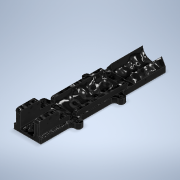
# Autodesk Inventor part: kicker_plate_modified
Saved by Autodesk Inventor 2020 (Build 240168000, 168)
## iProperties
Created: 2019-08-27
Part Number: kicker_plate_modified
Material: PET Plastic
Document SubType Name: Modeling
Designer: felip
Density: 1.541 g/cm^3
Appearance: Black
Author: felip
Autodesk Inventor part; units mm, degrees
ref_plane "YZ Plane" through (0, 0, 0) normal (1, 0, 0) x (0, 1, 0)
ref_plane "XZ Plane" through (0, 0, 0) normal (0, 1, 0) x (-1, 0, 0)
ref_plane "XY Plane" through (0, 0, 0) normal (0, 0, 1) x (1, 0, 0)
sketch "Sketch1" plane through (0, 0, 0) normal (0, 1, 0) x (-1, 0, 0)
  line L0 (0, 0) -> (29, 0)
  line L1 (29, 0) -> (29, -100)
  line L2 (29, -100) -> (0, -100)
  line L3 (0, -100) -> (0, 0)
  dimension "d0" = 29
  dimension "d1" = 100
  constraints: 8 end point, 2 parallel, 1 horizontal, 1 perpendicular
  measures "d0" distance of L1.end L2.end
  measures "d1" distance of L0.end L1.end
extrude "Extrusion1" add sketch "Sketch1" along normal blind 6
ref_plane "Work Plane1" through (-29, 0, -7) normal (0, 0, 1) x (1, 0, 0)
sketch "Sketch2" plane through (-29, 0, -7) normal (0, 0, 1) x (1, 0, 0)
  line L0 (0, 0) -> (29, 0) projected
  line L1 (29, 0) -> (29, 6) projected
  line L2 (0, 6) -> (29, 6) projected
  line L3 (0, 0) -> (0, 6) projected
  line L4 (29, 0) -> (0, 0) construction
  line L5 (14.5, 0) -> (14.5, 12.5) construction
  circle A0 centre (14.5, 12.5) radius 10.75
  point P0 (23.0623, 6)
  point P1 (5.9377, 6)
  dimension "d5" = 12.5
  dimension "d6" = 21.5
  constraints: 2 end point, 1 centre point, 1 coincident, 1 midpoint, 1 vertical
  measures "d5" distance of L5.start L5.end
  measures "d6" diameter of A0
extrude "Extrusion2" cut sketch "Sketch2" against normal blind 51.8 contours A0 L2 | L2 A0
sketch "Sketch9" plane through (0, 6, 0) normal (0, 1, 0) x (1, 0, 0)
  line L0 (-5.9377, 58.8) -> (-5.9377, 7) projected
  line L1 (-5.9377, 7) -> (-23.0623, 7) projected
  line L2 (-23.0623, 7) -> (-23.0623, 58.8) projected
  line L3 (-23.0623, 58.8) -> (-5.9377, 58.8) projected
  line L4 (-29, 100) -> (-29, 0) projected
  line L5 (-29, 0) -> (0, 0) projected
  line L6 (0, 0) -> (0, 100) projected
  line L7 (0, 100) -> (-29, 100) projected
  line L8 (-29, 100) -> (-29, 0) projected
  line L9 (0, 0) -> (0, 100) projected
  line L10 (-29, 100) -> (0, 100)
  line L11 (0, 100) -> (0, 66)
  line L12 (0, 66) -> (-29, 66)
  line L13 (-29, 66) -> (-29, 100)
  dimension "d60" = 34
  constraints: 8 end point, 2 parallel, 1 horizontal, 1 perpendicular, 1 point on line
  measures "d60" distance between parallel lines of L7 L12
extrude "Extrusion7" add sketch "Sketch9" along normal blind 6.75 contours L7 L6 L12 L4
sketch "Sketch3" plane through (0, 0, -100) normal (0, 0, -1) x (-1, 0, 0)
  line L0 (0, 0) -> (29, 0) projected
  line L1 (29, 0) -> (29, 12.75) projected
  line L2 (0, 0) -> (0, 12.75) projected
  line L3 (0, 0) -> (29, 0) construction
  line L4 (14.5, 0) -> (14.5, 12.5) construction
  circle A0 centre (14.5, 12.5) radius 10
  line L5 (0, 12.75) -> (29, 12.75) projected
  dimension "d9" = 12.5
  dimension "d10" = 20
  constraints: 2 end point, 1 centre point, 1 coincident, 1 midpoint, 1 vertical
  measures "d9" distance of L4.start L4.end
  measures "d10" diameter of A0
extrude "Extrusion3" cut sketch "Sketch3" against normal blind 34 contours L5 A0 | A0 L5
sketch "Sketch4" plane through (0, 0, 0) normal (0, -1, 0) x (1, 0, 0)
  line L0 (0, -100) -> (-29, -100) projected
  line L1 (0, 0) -> (0, -100) projected
  line L2 (-29, 0) -> (0, 0) projected
  line L3 (-29, -100) -> (-29, 0) projected
  point P0 (-24, -3)
  point P1 (-5, -3)
  point P2 (-24, -63)
  point P3 (-5, -63)
  dimension "d13" = 3
  dimension "d14" = 5
  dimension "d15" = 3
  dimension "d16" = 5
  dimension "d24" = 5
  dimension "d25" = 63
  dimension "d26" = 5
  dimension "d27" = 63
  measures "d13" distance from line of L2 point (-24, -3)
  measures "d14" distance from line of L3 point (-24, -3)
  measures "d15" distance from line of L2 point (-5, -3)
  measures "d16" distance from line of L1 point (-5, -3)
  measures "d24" distance from line of L3 point (-24, -63)
  measures "d25" distance from line of L2 point (-24, -63)
  measures "d26" distance from line of L1 point (-5, -63)
  measures "d27" distance from line of point (-5, -63) L2
hole "Hole1" at (-24, 0, -3) at (-5, 0, -3) at (-24, 0, -63) at (-5, 0, -63) direction (0, 1, 0) diameter 3.1 depth 6 counterbore diameter 5.5 counterbore depth 2
move faces "Move1" translate (0, 0, 31) faces at (-19.3333, 2, 0)
sketch "Sketch5" plane through (0, 6, 0) normal (0, 1, 0) x (1, 0, 0)
  circle A0 centre (-24, 63) radius 1.55 projected
  circle A1 centre (-24, 3) radius 1.55 projected
  circle A2 centre (-5, 3) radius 1.55 projected
  circle A3 centre (-5, 63) radius 1.55 projected
  line L0 (-6.9007, 66) -> (-22.0993, 66) projected
  line L1 (-29, 66) -> (-29, -31) projected
  line L2 (-29, -31) -> (0, -31) projected
  line L3 (0, -31) -> (0, 66) projected
  line L4 (-5.9377, 58.8) -> (-5.9377, 7) projected
  line L5 (-5.9377, 7) -> (-23.0623, 7) projected
  line L6 (-23.0623, 7) -> (-23.0623, 58.8) projected
  line L7 (-23.0623, 58.8) -> (-5.9377, 58.8) projected
  line L8 (-29, -31) -> (0, -31) projected
  line L9 (-9.25, -31) -> (-19.75, -31)
  line L10 (-19.75, -31) -> (-19.75, 0)
  line L11 (-19.75, 0) -> (-9.25, 0)
  line L12 (-9.25, 0) -> (-9.25, -31)
  line L13 (0, 66) -> (-6.9007, 66) projected
  line L14 (-22.0993, 66) -> (-29, 66) projected
  point P0 (0, 0)
  point P1 (-14.5, -31)
  point P2 (-9.25, -31)
  dimension "d31" = 10.5
  dimension "d32" = 31
  constraints: 8 end point, 2 midpoint, 2 parallel, 1 horizontal, 1 perpendicular, 1 point on line
  measures "d31" distance of L10.end L11.end
  measures "d32" distance of L9.end L10.end
extrude "Extrusion4" cut sketch "Sketch5" against normal blind 2.95 contours L2 L10 L11 L12
sketch "Sketch6" plane through (0, 6, 0) normal (0, 1, 0) x (1, 0, 0)
  line L0 (-5.9377, 58.8) -> (-5.9377, 7) projected
  line L1 (-5.9377, 7) -> (-23.0623, 7) projected
  line L2 (-23.0623, 7) -> (-23.0623, 58.8) projected
  line L3 (-23.0623, 58.8) -> (-5.9377, 58.8) projected
  line L4 (-19.75, -31) -> (-19.75, 0) projected
  line L5 (-19.75, 0) -> (-9.25, 0) projected
  line L6 (-9.25, 0) -> (-9.25, -31) projected
  line L7 (-9.25, -31) -> (0, -31) projected
  line L8 (0, -31) -> (0, 66) projected
  line L9 (-6.9007, 66) -> (-22.0993, 66) projected
  line L10 (-29, 66) -> (-29, -31) projected
  line L11 (-29, -31) -> (-19.75, -31) projected
  circle A0 centre (-5, 63) radius 1.55 projected
  circle A1 centre (-5, 3) radius 1.55 projected
  circle A2 centre (-24, 3) radius 1.55 projected
  circle A3 centre (-24, 63) radius 1.55 projected
  line L12 (-9.25, -31) -> (0, -31) projected
  line L13 (-2.125, -31) -> (-7.125, -31)
  line L14 (-7.125, -31) -> (-7.125, -11)
  line L15 (-7.125, -11) -> (-2.125, -11)
  line L16 (-2.125, -11) -> (-2.125, -31)
  line L17 (-21.875, -31) -> (-26.875, -31)
  line L18 (-26.875, -31) -> (-26.875, -11)
  line L19 (-26.875, -11) -> (-21.875, -11)
  line L20 (-21.875, -11) -> (-21.875, -31)
  line L21 (0, 66) -> (-6.9007, 66) projected
  line L22 (-22.0993, 66) -> (-29, 66) projected
  line L23 (-19.75, -31) -> (-19.75, 0) projected
  line L24 (-21.875, 0) -> (-19.75, 0)
  line L25 (-19.75, 0) -> (-19.75, -31)
  line L26 (-19.75, -31) -> (-21.875, -31)
  line L27 (-21.875, -31) -> (-21.875, 0)
  line L28 (-9.25, 0) -> (-9.25, -31) projected
  line L29 (-7.125, 0) -> (-9.25, 0)
  line L30 (-9.25, 0) -> (-9.25, -31)
  line L31 (-9.25, -31) -> (-7.125, -31)
  line L32 (-7.125, -31) -> (-7.125, 0)
  point P0 (0, 0)
  point P1 (-4.625, -31)
  point P2 (-24.375, -31)
  point P3 (-26.875, -31)
  point P4 (-2.125, -31)
  dimension "d35" = 5
  dimension "d36" = 20
  dimension "d37" = 5
  dimension "d38" = 20
  constraints: 32 end point, 8 parallel, 4 horizontal, 4 midpoint, 4 perpendicular, 3 point on line
  measures "d35" distance of L14.end L15.end
  measures "d36" distance of L13.end L14.end
  measures "d37" distance of L18.end L19.end
  measures "d38" distance of L17.end L18.end
extrude "Extrusion5" add sketch "Sketch6" along normal blind 14 contours L11 L18 L19 L20 | L14 L15 L16 L7
sketch "Sketch7" plane through (0, 0, 0) normal (0, -1, 0) x (1, 0, 0)
  circle A0 centre (-24, -63) radius 2.75 projected
  circle A1 centre (-24, -3) radius 2.75 projected
  circle A2 centre (-5, -3) radius 2.75 projected
  circle A3 centre (-5, -63) radius 2.75 projected
  line L0 (0, -100) -> (-29, -100) projected
  line L1 (0, 31) -> (0, -100) projected
  line L2 (-29, 31) -> (0, 31) projected
  line L3 (-29, -100) -> (-29, 31) projected
  line L4 (-29, -100) -> (-29, 31) construction
  line L5 (0, 31) -> (0, -100) construction
  line L6 (-29, -100) -> (-29, 31) projected
  line L7 (-29, -52) -> (-36, -52)
  line L8 (-36, -52) -> (-36, -45)
  line L9 (-36, -45) -> (-29, -45)
  line L10 (-29, -45) -> (-29, -52)
  line L11 (-29, -7) -> (-36, -7)
  line L12 (-36, -7) -> (-36, 0)
  line L13 (-36, 0) -> (-29, 0)
  line L14 (-29, 0) -> (-29, -7)
  line L15 (-4.5, -100) -> (-24.5, -100) construction
  line L16 (-14.5, -100) -> (-14.5, 31) construction
  line L17 (-29, 31) -> (0, 31) construction
  line L18 (0, -52) -> (7, -52)
  line L19 (7, -52) -> (7, -45)
  line L20 (7, -45) -> (0, -45)
  line L21 (0, -45) -> (0, -52)
  line L22 (0, -7) -> (7, -7)
  line L23 (7, -7) -> (7, 0)
  line L24 (7, 0) -> (0, 0)
  line L25 (0, 0) -> (0, -7)
  point P0 (0, 0)
  point P1 (0, 0)
  point P2 (0, -7)
  point P3 (0, -45)
  point P4 (0, -52)
  point P5 (-29, 0)
  point P6 (-24.4969, -100)
  point P7 (-4.5031, -100)
  dimension "d41" = 7
  dimension "d42" = 7
  dimension "d43" = 7
  dimension "d44" = 7
  dimension "d58" = 31
  dimension "d59" = 38
  constraints: 34 end point, 8 symmetric about line, 4 parallel, 2 horizontal, 2 midpoint, 2 perpendicular, 2 point on line
  measures "d41" distance of L8.end L9.end
  measures "d42" distance of L7.end L8.end
  measures "d43" distance of L12.end L13.end
  measures "d44" distance of L11.end L12.end
  measures "d58" distance between parallel lines of L13 L2
  measures "d59" distance between parallel lines of L9 L11
extrude "Extrusion6" add sketch "Sketch7" against normal blind 6 contours L1 L20 L19 L18 | L7 L8 L9 L3 | L1 L24 L23 L22 | L11 L12 L13 L3
sketch "Sketch8" plane through (0, 0, 0) normal (0, -1, 0) x (1, 0, 0)
  circle A0 centre (-24, -63) radius 2.75 projected
  circle A1 centre (-24, -3) radius 2.75 projected
  circle A2 centre (-5, -3) radius 2.75 projected
  circle A3 centre (-5, -63) radius 2.75 projected
  line L0 (-29, 31) -> (0, 31) projected
  line L1 (-29, 0) -> (-29, 31) projected
  line L2 (-29, 0) -> (-36, 0) projected
  line L3 (-36, 0) -> (-36, -7) projected
  line L4 (-36, -7) -> (-29, -7) projected
  line L5 (-29, -45) -> (-29, -7) projected
  line L6 (-29, -45) -> (-36, -45) projected
  line L7 (-36, -45) -> (-36, -52) projected
  line L8 (-36, -52) -> (-29, -52) projected
  line L9 (-29, -100) -> (-29, -52) projected
  line L10 (0, -100) -> (-29, -100) projected
  line L11 (0, -52) -> (0, -100) projected
  line L12 (0, -52) -> (7, -52) projected
  line L13 (7, -52) -> (7, -45) projected
  line L14 (7, -45) -> (0, -45) projected
  line L15 (0, -7) -> (0, -45) projected
  line L16 (0, -7) -> (7, -7) projected
  line L17 (7, -7) -> (7, 0) projected
  line L18 (7, 0) -> (0, 0) projected
  line L19 (0, 31) -> (0, 0) projected
  line L20 (7, -52) -> (7, -45) construction
  line L21 (7, -48.5) -> (-36, -48.5) construction
  line L22 (-36, -52) -> (-36, -45) construction
  line L23 (7, -7) -> (7, 0) construction
  line L24 (7, -3.5) -> (-36, -3.5) construction
  point P0 (0, 0)
  point P1 (3.5, -48.5)
  point P2 (-32.5, -48.5)
  point P3 (-32.5, -3.5)
  point P4 (3.5, -3.5)
  dimension "d47" = 3.5
  dimension "d48" = 3.5
  dimension "d49" = 3.5
  dimension "d50" = 3.5
  constraints: 4 end point, 4 midpoint, 4 point on line
  measures "d47" distance from line of L13 point (3.5, -48.5)
  measures "d48" distance from line of L7 point (-32.5, -48.5)
  measures "d49" distance from line of L3 point (-32.5, -3.5)
  measures "d50" distance from line of L17 point (3.5, -3.5)
hole "Hole2" at (3.5, 0, -48.5) at (-32.5, 0, -48.5) at (-32.5, 0, -3.5) at (3.5, 0, -3.5) direction (0, 1, 0) diameter 3.1 depth 6 counterbore diameter 5.5 counterbore depth 2
sketch "Sketch10" plane through (0, 0, 0) normal (0, -1, 0) x (1, 0, 0)
  circle A0 centre (-32.5, -3.5) radius 2.75 projected
  circle A1 centre (3.5, -48.5) radius 2.75 projected
  circle A2 centre (-32.5, -48.5) radius 2.75 projected
  circle A3 centre (3.5, -3.5) radius 2.75 projected
  circle A4 centre (-24, -63) radius 2.75 projected
  circle A5 centre (-24, -3) radius 2.75 projected
  circle A6 centre (-5, -3) radius 2.75 projected
  circle A7 centre (-5, -63) radius 2.75 projected
  line L0 (-29, -100) -> (-29, -52) projected
  line L1 (0, -100) -> (-29, -100) projected
  line L2 (0, -52) -> (0, -100) projected
  line L3 (0, -52) -> (7, -52) projected
  line L4 (7, -52) -> (7, -45) projected
  line L5 (7, -45) -> (0, -45) projected
  line L6 (0, -7) -> (0, -45) projected
  line L7 (0, -7) -> (7, -7) projected
  line L8 (7, -7) -> (7, 0) projected
  line L9 (7, 0) -> (0, 0) projected
  line L10 (0, 31) -> (0, 0) projected
  line L11 (-29, 31) -> (0, 31) projected
  line L12 (-29, 0) -> (-29, 31) projected
  line L13 (-29, 0) -> (-36, 0) projected
  line L14 (-36, 0) -> (-36, -7) projected
  line L15 (-36, -7) -> (-29, -7) projected
  line L16 (-29, -45) -> (-29, -7) projected
  line L17 (-29, -45) -> (-36, -45) projected
  line L18 (-36, -45) -> (-36, -52) projected
  line L19 (-36, -52) -> (-29, -52) projected
  line L20 (-29, 31) -> (0, 31) construction
  line L21 (-14.5, 31) -> (-14.5, -24) construction
  circle A8 centre (-14.5, -24) radius 88
  circle A9 centre (-14.5, -24) radius 76
  point P0 (0, 0)
  point P1 (-14.5, -100)
  point P2 (-29, -98.604)
  point P3 (0, -98.604)
  dimension "d63" = 55
  dimension "d64" = 176
  dimension "d65" = 152
  constraints: 2 centre point, 2 coincident, 2 end point, 1 midpoint, 1 vertical
  measures "d63" distance of L21.start L21.end
  measures "d64" diameter of A8
  measures "d65" diameter of A9
extrude "Extrusion8" cut sketch "Sketch10" against normal blind 85.25 contours L0 A9 L1 | A9 L2 L1
fillet "Fillet1" radius 1 8 edges at (-2.125, 6, 21) (0, 6, 15.5) (-7.125, 6, 21) (-9.25, 6, 15.5) (-19.75, 6, 15.5) (-21.875, 6, 21) (-26.875, 6, 21) (-29, 6, 15.5)
fillet "Fillet1" radius 3 2 edges at (-4.625, 20, 11) (-24.375, 20, 11)
fillet "Fillet2" radius 3 10 edges at (-29, 3, -52) (-29, 3, -45) (-29, 3, -7) (-28.7071, 5.7071, 0) (-29, 2.5, 0) (-0.2929, 5.7071, 0) (0, 2.5, 0) (0, 3, -7) (0, 3, -52) (0, 3, -45)
fillet "Fillet2" radius 3 8 edges at (7, 3, -45) (7, 3, -52) (7, 3, 0) (7, 3, -7) (-36, 3, 0) (-36, 3, -7) (-36, 3, -45) (-36, 3, -52)
fillet "Fillet3" radius 1 39 edges at (-29.8787, 0, -52.8787) (-32.5, 0, -52) (-35.1213, 0, -51.1213) (-36, 0, -48.5) (-35.1213, 0, -45.8787) (-32.5, 0, -45) (-29.8787, 0, -44.1213) (-29, 0, -26) (-29.8787, 0, -7.8787) (-32.5, 0, -7) (-35.1213, 0, -6.1213) (-36, 0, -3.5) (-35.1213, 0, -0.8787) (-32.5, 0, 0) (-29.8787, 0, 0.8787) (-29, 0, 17) (-29, 0, -76.802) (0.8787, 0, -52.8787) (3.5, 0, -52) (6.1213, 0, -51.1213) (7, 0, -48.5) (6.1213, 0, -45.8787) (3.5, 0, -45) (0.8787, 0, -44.1213) (0, 0, -26) (0.8787, 0, -7.8787) (3.5, 0, -7) (6.1213, 0, -6.1213) (7, 0, -3.5) (6.1213, 0, -0.8787) (3.5, 0, 0) (0.8787, 0, 0.8787) (0, 0, 17) (0, 0, -76.802) (-14.5, 0, -100) (-24, 0, -60.25) (-5, 0, -60.25) (-5, 0, -0.25) (-24, 0, -0.25)
chamfer "Chamfer1" distance 4.5 distance2 6 1 edges at (-29, 12.75, -82.302) measured on face at (-28.5, 12.75, -82.302)
chamfer "Chamfer2" distance 4.5 distance2 6 1 edges at (0, 12.75, -82.302) measured on face at (-0.5, 12.75, -82.302)
fillet "Fillet4" [suppressed]
sketch "Sketch11" plane through (-19.75, 3.05, 31) normal (0, 0, 1) x (1, 0, 0)
  arc A0 (18.75, -3.05) -> (19.75, -2.05) centre (18.75, -2.05) ccw projected
  line L0 (19.75, -2.05) -> (19.75, 1.95) projected
  arc A1 (19.75, 1.95) -> (18.75, 2.95) centre (18.75, 1.95) ccw projected
  line L1 (18.625, 2.95) -> (18.75, 2.95) projected
  arc A2 (17.625, 3.95) -> (18.625, 2.95) centre (18.625, 3.95) ccw projected
  line L2 (17.625, 3.95) -> (17.625, 16.95) projected
  line L3 (12.625, 16.95) -> (17.625, 16.95) projected
  line L4 (12.625, 3.95) -> (12.625, 16.95) projected
  arc A3 (11.625, 2.95) -> (12.625, 3.95) centre (11.625, 3.95) ccw projected
  line L5 (11.5, 2.95) -> (11.625, 2.95) projected
  arc A4 (11.5, 2.95) -> (10.5, 1.95) centre (11.5, 1.95) ccw projected
  line L6 (10.5, 1.95) -> (10.5, 0) projected
  line L7 (10.5, 0) -> (0, 0) projected
  line L8 (0, 0) -> (0, 1.95) projected
  arc A5 (0, 1.95) -> (-1, 2.95) centre (-1, 1.95) ccw projected
  line L9 (-1.125, 2.95) -> (-1, 2.95) projected
  arc A6 (-2.125, 3.95) -> (-1.125, 2.95) centre (-1.125, 3.95) ccw projected
  line L10 (-2.125, 3.95) -> (-2.125, 16.95) projected
  line L11 (-7.125, 16.95) -> (-2.125, 16.95) projected
  line L12 (-7.125, 3.95) -> (-7.125, 16.95) projected
  arc A7 (-8.125, 2.95) -> (-7.125, 3.95) centre (-8.125, 3.95) ccw projected
  line L13 (-8.25, 2.95) -> (-8.125, 2.95) projected
  arc A8 (-8.25, 2.95) -> (-9.25, 1.95) centre (-8.25, 1.95) ccw projected
  line L14 (-9.25, -2.05) -> (-9.25, 1.95) projected
  arc A9 (-9.25, -2.05) -> (-8.25, -3.05) centre (-8.25, -2.05) ccw projected
  line L15 (-8.25, -3.05) -> (18.75, -3.05) projected
  point P0 (19.75, -3.05)
extrude "Extrusion9" add sketch "Sketch11" along normal blind 1.45
fillet "Fillet5" radius 3 2 edges at (-4.625, 20, 32.45) (-24.375, 20, 32.45)
fillet "Fillet5" radius 1 13 edges at (-0.2929, 0.2929, 32.45) (0, 3, 32.45) (-0.2929, 5.7071, 32.45) (-1.0625, 6, 32.45) (-1.8321, 6.2929, 32.45) (-2.125, 13.5, 32.45) (-28.7071, 0.2929, 32.45) (-29, 3, 32.45) (-28.7071, 5.7071, 32.45) (-27.9375, 6, 32.45) (-27.1679, 6.2929, 32.45) (-26.875, 13.5, 32.45) (-14.5, 0, 32.45)
sketch "Sketch12" plane through (0, 6, 0) normal (0, 1, 0) x (1, 0, 0)
  line L0 (-0.9, 6.1) -> (-28.1, 6.1)
  line L1 (-28.1, 6.1) -> (-28.1, 59.9)
  line L2 (-28.1, 59.9) -> (-0.9, 59.9)
  line L3 (-0.9, 59.9) -> (-0.9, 6.1)
  line L4 (-23.0623, 7) -> (-23.0623, 58.8) projected
  line L5 (-23.0623, 7) -> (-5.9377, 7) projected
  line L6 (-5.9377, 58.8) -> (-5.9377, 7) projected
  line L7 (-5.9377, 58.8) -> (-23.0623, 58.8) projected
  line L8 (-7.125, -11) -> (-7.125, -14) projected
  line L9 (-7.125, -14) -> (-2.125, -14) projected
  line L10 (-2.125, -14) -> (-2.125, -11) projected
  line L11 (-2.125, -11) -> (-7.125, -11) projected
  line L12 (-26.875, -11) -> (-26.875, -14) projected
  line L13 (-26.875, -14) -> (-21.875, -14) projected
  line L14 (-21.875, -14) -> (-21.875, -11) projected
  line L15 (-21.875, -11) -> (-26.875, -11) projected
  line L16 (-2.125, -11) -> (-7.125, -11)
  line L17 (-7.125, -11) -> (-7.125, -0.1)
  line L18 (-7.125, -0.1) -> (-2.125, -0.1)
  line L19 (-2.125, -0.1) -> (-2.125, -11)
  line L20 (-21.875, -11) -> (-26.875, -11)
  line L21 (-26.875, -11) -> (-26.875, -0.1)
  line L22 (-26.875, -0.1) -> (-21.875, -0.1)
  line L23 (-21.875, -0.1) -> (-21.875, -11)
  point P0 (0, 0)
  point P1 (-14.5, 6.1)
  dimension "d84" = 6.1
  dimension "d85" = 27.2
  dimension "d87" = 14.5
  dimension "d88" = 53.8
  dimension "d89" = 0.1
  dimension "d90" = 0.1
  constraints: 24 end point, 6 parallel, 3 horizontal, 3 perpendicular, 1 midpoint
  measures "d84" distance from line of point (0, 0) L0
  measures "d85" distance between parallel lines of L1 L3
  measures "d87" horizontal distance of point (0, 0) point (-14.5, 6.1)
  measures "d88" distance between parallel lines of L2 L0
  measures "d89" distance from line of L18 point (0, 0)
  measures "d90" distance from line of L22 point (0, 0)
extrude "Extrusion10" add sketch "Sketch12" along normal blind 5 contours L0 L1 L2 L3 | L4 L7 L6 L5 | L17 L18 L19 L11 | L21 L22 L23 L15
extrude "Extrusion11" cut sketch "Sketch2" along normal blind 5 and the other way blind 53.75 contours A0 L2 picked at (13.7572, 12.4667)
sketch "Sketch14" plane through (0, 0, 0) normal (0, -1, 0) x (1, 0, 0)
  line L0 (-29.4397, -71.5814) -> (0, -71.5814)
  line L1 (0, -71.5814) -> (0, -112.0692)
  line L2 (0, -112.0692) -> (-29.4397, -112.0692)
  line L3 (-29.4397, -112.0692) -> (-29.4397, -71.5814)
  point P0 (0, 0)
  constraints: 8 end point, 2 parallel, 1 horizontal, 1 perpendicular
extrude "Extrusion12" [suppressed]
sketch "Sketch16" plane through (0, 20, 0) normal (0, 1, 0) x (1, 0, 0)
  line L0 (-9.25, 0) -> (-9.25, -32.45) projected
  line L1 (-19.75, 0) -> (-9.25, 0) projected
  line L2 (-19.75, -32.45) -> (-19.75, 0) projected
  line L3 (-9.25, -32.45) -> (-19.75, -32.45) projected
  line L4 (-21.875, -14) -> (-21.875, -29.45) projected
  line L5 (-7.125, -14) -> (-7.125, -29.45) projected
  line L6 (-1, -32.45) -> (-28, -32.45) projected
  line L7 (-21.875, -32.45) -> (-7.125, -32.45)
  line L8 (-7.125, -32.45) -> (-7.125, -14)
  line L9 (-7.125, -14) -> (-21.875, -14)
  line L10 (-21.875, -14) -> (-21.875, -32.45)
  point P0 (0, 0)
  point P1 (-19.75, -14)
  point P2 (-9.25, -14)
  constraints: 8 end point, 2 parallel, 1 horizontal, 1 perpendicular, 1 point on line
extrude "Extrusion13" cut sketch "Sketch16" against normal up to surface (16.95 mm away)
fillet "Fillet6" radius 2 6 edges at (-26.6224, 11, -6.1) (-24.375, 11, 0.1) (-4.625, 11, 0.1) (-2.3776, 11, -6.1) (-2.3776, 11, -59.9) (-26.6224, 11, -59.9)
sketch "Sketch17" plane through (-0.9, 6, -6.1) normal (1, 0, 0) x (0, 0, -1)
  arc A0 (53.8, 3) -> (51.8, 5) centre (51.8, 3) ccw projected
  line L0 (2, 5) -> (51.8, 5) projected
  arc A1 (2, 5) -> (0, 3) centre (2, 3) ccw projected
  line L1 (0, 0) -> (0, 3) projected
  line L2 (53.8, 0) -> (0, 0) projected
  line L3 (53.8, 0) -> (53.8, 3) projected
  line L4 (93.2392, 6.75) -> (59.9, 6.75) projected
  line L5 (59.9, 6.75) -> (59.9, 0.75) projected
  line L6 (59.9, 0.75) -> (92.504, 0.75) projected
  arc A2 (-6.2, 3) -> (-8.2, 5) centre (-8.2, 3) ccw projected
  line L7 (-17.1, 5) -> (-8.2, 5) projected
  line L8 (-17.1, 5) -> (-17.1, 11) projected
  arc A3 (-17.1, 11) -> (-20.1, 14) centre (-20.1, 11) ccw projected
  line L9 (-20.1, 14) -> (-35.55, 14) projected
  arc A4 (-35.55, 14) -> (-37.55, 13.2361) centre (-35.55, 11) ccw projected
  line L10 (-37.55, 1) -> (-37.55, 13.2361) projected
  line L11 (-17.1, 1) -> (-37.55, 1) projected
  line L12 (-6.2, 0) -> (-17.1, 0) projected
  line L13 (-6.2, 0) -> (-6.2, 3) projected
  line L14 (-6.2, 0) -> (-17.1, 0) projected
  line L15 (-6.35, 0) -> (0.15, 0)
  line L16 (0.15, 0) -> (0.15, 5)
  line L17 (0.15, 5) -> (-6.35, 5)
  line L18 (-6.35, 5) -> (-6.35, 0)
  line L19 (53.65, 0) -> (60.05, 0)
  line L20 (60.05, 0) -> (60.05, 6.75)
  line L21 (60.05, 6.75) -> (53.65, 6.75)
  line L22 (53.65, 6.75) -> (53.65, 0)
  line L23 (-17.1, 0) -> (-17.1, 1) projected
  ellipse E0 centre (17.9, 20.0833) end of major axis (17.9, 121.4167) minor radius 76 (92.504, 0.75) -> (93.2392, 6.75) ccw projected
  point P0 (-6.1, -6)
  point P1 (60.05, 0.75)
  point P2 (53.65, 3.7599)
  point P3 (-6.35, 3.7599)
  point P4 (0.15, 3.7599)
  dimension "d103" = 0.15
  dimension "d104" = 0.15
  dimension "d105" = 0.15
  dimension "d106" = 0.15
  dimension "d107" = 0
  constraints: 16 end point, 4 parallel, 2 horizontal, 2 perpendicular, 1 point on line, 1 other
  measures "d103" distance between parallel lines of L13 L18
  measures "d104" distance between parallel lines of L1 L16
  measures "d105" distance between parallel lines of L3 L22
  measures "d106" distance between parallel lines of L5 L20
  measures "d107" distance between parallel lines of L4 L21
extrude "Extrusion14" cut sketch "Sketch17" against normal up to surface (28.1 mm away) contours A0 L22 L21 L5 L6 L20 L19 L3 | A1 L1 L15 L13 A2 L18 L17 L16
sketch "Sketch18" plane through (0, 2.75, 0) normal (0, 1, 0) x (1, 0, 0)
  line L0 (-9.125, -14) -> (-9.125, -32) projected
  line L1 (-9.25, -14) -> (-9.125, -14) projected
  line L2 (-19.875, -14) -> (-19.75, -14) projected
  line L3 (-19.875, -32) -> (-19.875, -14) projected
  line L4 (-9.125, -32) -> (-9.25, -32) projected
  line L5 (-20.75, -14) -> (-19.75, -14) projected
  line L6 (-19.75, -14) -> (-19.75, 0) projected
  line L7 (-19.75, 0) -> (-20.75, 0) projected
  line L8 (-20.75, 0) -> (-20.75, -14) projected
  line L9 (-29, 66.15) -> (-29, 55) projected
  arc A0 (-32, 52) -> (-29, 55) centre (-32, 55) ccw projected
  line L10 (-32, 52) -> (-33, 52) projected
  arc A1 (-33, 52) -> (-36, 49) centre (-33, 49) ccw projected
  line L11 (-36, 49) -> (-36, 48) projected
  arc A2 (-36, 48) -> (-33, 45) centre (-33, 48) ccw projected
  line L12 (-33, 45) -> (-32, 45) projected
  arc A3 (-29, 42) -> (-32, 45) centre (-32, 42) ccw projected
  line L13 (-29, 42) -> (-29, 10) projected
  arc A4 (-32, 7) -> (-29, 10) centre (-32, 10) ccw projected
  line L14 (-32, 7) -> (-33, 7) projected
  arc A5 (-33, 7) -> (-36, 4) centre (-33, 4) ccw projected
  line L15 (-36, 4) -> (-36, 3) projected
  arc A6 (-36, 3) -> (-33, 0) centre (-33, 3) ccw projected
  line L16 (-33, 0) -> (-31.873, 0) projected
  line L17 (-28, -3) -> (-28, -31.45) projected
  line L18 (-27.875, -31.45) -> (-28, -31.45) projected
  line L19 (-27.875, -11) -> (-27.875, -31.45) projected
  line L20 (-27.875, -11) -> (-26.875, -11) projected
  line L21 (-26.875, -11) -> (-26.875, -0.1) projected
  line L22 (-26.875, -0.1) -> (-21.875, -0.1) projected
  line L23 (-21.875, -0.1) -> (-21.875, -11) projected
  line L24 (-21.875, -11) -> (-20.875, -11) projected
  line L25 (-20.875, -11) -> (-20.875, -14) projected
  line L26 (-20.875, -14) -> (-20.75, -14) projected
  line L27 (-20.75, 0) -> (-20.75, -14) projected
  line L28 (-20.75, 0) -> (-8.25, 0) projected
  line L29 (-8.25, 0) -> (-8.25, -14) projected
  line L30 (-8.25, -14) -> (-8.125, -14) projected
  line L31 (-8.125, -11) -> (-8.125, -14) projected
  line L32 (-8.125, -11) -> (-7.125, -11) projected
  line L33 (-7.125, -11) -> (-7.125, -0.1) projected
  line L34 (-7.125, -0.1) -> (-2.125, -0.1) projected
  line L35 (-2.125, -0.1) -> (-2.125, -11) projected
  line L36 (-2.125, -11) -> (-1.125, -11) projected
  line L37 (-1.125, -11) -> (-1.125, -31.45) projected
  line L38 (-1, -31.45) -> (-1.125, -31.45) projected
  line L39 (-1, -3) -> (-1, -31.45) projected
  line L40 (2.873, 0) -> (4, 0) projected
  arc A7 (4, 0) -> (7, 3) centre (4, 3) ccw projected
  line L41 (7, 3) -> (7, 4) projected
  arc A8 (7, 4) -> (4, 7) centre (4, 4) ccw projected
  line L42 (4, 7) -> (3, 7) projected
  arc A9 (0, 10) -> (3, 7) centre (3, 10) ccw projected
  line L43 (0, 10) -> (0, 42) projected
  arc A10 (3, 45) -> (0, 42) centre (3, 42) ccw projected
  line L44 (3, 45) -> (4, 45) projected
  arc A11 (4, 45) -> (7, 48) centre (4, 48) ccw projected
  line L45 (7, 48) -> (7, 49) projected
  arc A12 (7, 49) -> (4, 52) centre (4, 49) ccw projected
  line L46 (4, 52) -> (3, 52) projected
  arc A13 (0, 55) -> (3, 52) centre (3, 55) ccw projected
  line L47 (0, 55) -> (0, 66) projected
  line L48 (0, 66) -> (-0.9, 66) projected
  line L49 (-0.9, 66) -> (-0.9, 66.15) projected
  line L50 (-0.9, 66.15) -> (-6.9007, 66.15) projected
  line L51 (-6.9007, 66) -> (-6.9007, 66.15) projected
  line L52 (-6.9007, 66) -> (-22.0993, 66) projected
  line L53 (-22.0993, 66.15) -> (-22.0993, 66) projected
  line L54 (-22.0993, 66.15) -> (-29, 66.15) projected
  circle A14 centre (3.5, 3.5) radius 1.55 projected
  circle A15 centre (3.5, 48.5) radius 1.55 projected
  circle A16 centre (-32.5, 3.5) radius 1.55 projected
  circle A17 centre (-32.5, 48.5) radius 1.55 projected
  circle A18 centre (-5, 3) radius 1.55 projected
  circle A19 centre (-24, 3) radius 1.55 projected
  circle A20 centre (-24, 63) radius 1.55 projected
  circle A21 centre (-5, 63) radius 1.55 projected
  line L55 (-28.1, 59.9) -> (-23.0623, 59.9) projected
  line L56 (-23.0623, 59.9) -> (-23.0623, 58.8) projected
  line L57 (-23.0623, 58.8) -> (-5.9377, 58.8) projected
  line L58 (-5.9377, 58.8) -> (-5.9377, 59.9) projected
  line L59 (-5.9377, 59.9) -> (-0.9, 59.9) projected
  line L60 (-0.9, 59.9) -> (-0.9, 6.1) projected
  line L61 (-0.9, 6.1) -> (-5.9377, 6.1) projected
  line L62 (-5.9377, 6.1) -> (-5.9377, 7) projected
  line L63 (-5.9377, 7) -> (-23.0623, 7) projected
  line L64 (-23.0623, 7) -> (-23.0623, 6.1) projected
  line L65 (-23.0623, 6.1) -> (-28.1, 6.1) projected
  line L66 (-28.1, 6.1) -> (-28.1, 59.9) projected
  line L67 (-9.25, -14) -> (-8.25, -14) projected
  line L68 (-8.25, 0) -> (-8.25, -14) projected
  line L69 (-8.25, 0) -> (-9.25, 0) projected
  line L70 (-9.25, 0) -> (-9.25, -14) projected
  line L71 (-9.125, -14) -> (-7.125, -14) projected
  line L72 (-9.125, -14) -> (-9.125, -32) projected
  line L73 (-9.125, -32) -> (-7.125, -32) projected
  line L74 (-7.125, -32) -> (-7.125, -14) projected
  line L75 (-1, -32) -> (-28, -32) projected
  line L76 (-21.875, -0.1) -> (-19.75, -0.1)
  line L77 (-19.75, -0.1) -> (-19.75, -32)
  line L78 (-19.75, -32) -> (-21.875, -32)
  line L79 (-21.875, -32) -> (-21.875, -0.1)
  line L80 (-7.125, 4) -> (-9.25, 4)
  line L81 (-9.25, 4) -> (-9.25, -32)
  line L82 (-9.25, -32) -> (-7.125, -32)
  line L83 (-7.125, -32) -> (-7.125, 4)
  line L84 (-21.875, -0.1) -> (-21.875, 0)
  line L85 (-21.875, 0) -> (-19.75, 0)
  line L86 (-19.75, 0) -> (-19.75, -0.1)
  line L87 (-19.75, -0.1) -> (-21.875, -0.1)
  line L88 (-21.875, -0.1) -> (-21.875, 0)
  line L89 (-9.25, -32) -> (-9.25, -14) projected
  line L90 (-19.75, -32) -> (-19.875, -32) projected
  line L91 (-19.75, -14) -> (-19.75, -32) projected
  point P0 (0, 0)
  point P1 (-7.125, -0.1)
  point P2 (-8.25, 0)
  point P3 (-9.25, -14)
  point P4 (-9.25, 0)
  constraints: 26 end point, 6 parallel, 3 horizontal, 3 perpendicular, 2 point on line, 1 vertical, 2 other
extrude "Extrusion15" [suppressed]
fillet "Fillet7" [suppressed]
fillet "Fillet8" [suppressed]
sketch "Sketch19" plane through (-8.25, 6, 14) normal (0, 0, 1) x (1, 0, 0)
  line L0 (1.125, 1) -> (1.125, -2.95) projected
  arc A0 (0.125, 0) -> (1.125, 1) centre (0.125, 1) ccw projected
  line L1 (0, 0) -> (0.125, 0) projected
  arc A1 (0, 0) -> (-1, -1) centre (0, -1) ccw projected
  line L2 (-1, -2.95) -> (-1, -1) projected
  line L3 (-11.5, -1) -> (-11.5, -2.95) projected
  arc A2 (-11.5, -1) -> (-12.5, 0) centre (-12.5, -1) ccw projected
  line L4 (-12.625, 0) -> (-12.5, 0) projected
  arc A3 (-13.625, 1) -> (-12.625, 0) centre (-12.625, 1) ccw projected
  line L5 (-13.625, 1) -> (-13.625, -2.95) projected
  line L6 (1.125, 1) -> (1.125, -2.95) projected
  arc A4 (0.125, 0) -> (1.125, 1) centre (0.125, 1) ccw projected
  line L7 (0, 0) -> (0.125, 0) projected
  arc A5 (0, 0) -> (-1, -1) centre (0, -1) ccw projected
  line L8 (-1, -2.95) -> (-1, -1) projected
  line L9 (1.125, -2.95) -> (-1, -2.95) projected
  line L10 (1.125, -2.95) -> (-1, -2.95) projected
  line L11 (-11.5, -2.95) -> (-13.625, -2.95) projected
  point P0 (8.25, -6)
extrude "Extrusion16" cut sketch "Sketch19" against normal up to surface (14 mm away)
fillet "Fillet9" radius 2 2 edges at (-21.875, 3.05, 16.225) (-7.125, 3.05, 16.225)
equation "\"d48\" = d47"
equation "\"d49\" = d47"
equation "\"d50\" = d47"
body "Solid1"
